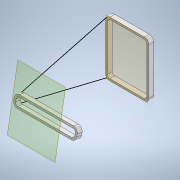
# Autodesk Inventor part: Rear Fan Shrowd
Saved by Autodesk Inventor 2020 (Build 240168000, 168)
## iProperties
Created: 2019-09-23
Part Number: Rear Fan Shrowd
Material: Generic
Document SubType Name: Modeling
Designer: pepd9
Density: 1 g/cm^3
Appearance: Default
Author: pepd9
Autodesk Inventor part; units mm, degrees
ref_plane "YZ Plane" through (0, 0, 0) normal (1, 0, 0) x (0, 1, 0)
ref_plane "XZ Plane" through (0, 0, 0) normal (0, 1, 0) x (-1, 0, 0)
ref_plane "XY Plane" through (0, 0, 0) normal (0, 0, 1) x (1, 0, 0)
ref_plane "Work Plane1" through (0, 0, 0) normal (0, 0, 1) x (1, 0, 0)
sketch "Sketch1" plane through (0, 0, 0) normal (0, 0, 1) x (1, 0, 0)
  line L0 (15.4, -2) -> (15.4, -18.2) projected
  arc A0 (15.4, -2) -> (13.4, 0) centre (13.4, -2) ccw projected
  line L1 (2, 0) -> (13.4, 0) projected
  arc A1 (2, 0) -> (0, -2) centre (2, -2) ccw projected
  line L2 (0, -18.2) -> (0, -2) projected
  arc A2 (0, -18.2) -> (2, -20.2) centre (2, -18.2) ccw projected
  line L3 (2, -20.2) -> (13.4, -20.2) projected
  arc A3 (13.4, -20.2) -> (15.4, -18.2) centre (13.4, -18.2) ccw projected
  arc A4 (1, -18.2) -> (2, -19.2) centre (2, -18.2) ccw projected
  line L4 (1, -2) -> (1, -18.2) projected
  arc A5 (2, -1) -> (1, -2) centre (2, -2) ccw projected
  line L5 (2, -1) -> (13.4, -1) projected
  arc A6 (14.4, -2) -> (13.4, -1) centre (13.4, -2) ccw projected
  line L6 (14.4, -2) -> (14.4, -18.2) projected
  arc A7 (13.4, -19.2) -> (14.4, -18.2) centre (13.4, -18.2) ccw projected
  line L7 (2, -19.2) -> (13.4, -19.2) projected
  line L8 (0.7, -20.5) -> (14.7, -20.5)
  line L9 (15.7, -19.5) -> (15.7, -0.7)
  line L10 (14.7, 0.3) -> (0.7, 0.3)
  line L11 (-0.3, -0.7) -> (-0.3, -19.5)
  arc A8 (0.7, 0.3) -> (-0.3, -0.7) centre (0.7, -0.7) ccw
  arc A9 (15.7, -0.7) -> (14.7, 0.3) centre (14.7, -0.7) ccw
  arc A10 (14.7, -20.5) -> (15.7, -19.5) centre (14.7, -19.5) ccw
  arc A11 (-0.3, -19.5) -> (0.7, -20.5) centre (0.7, -19.5) ccw
  line L12 (-1.1, -19.5) -> (-1.1, -0.7)
  arc A12 (0.7, 1.1) -> (-1.1, -0.7) centre (0.7, -0.7) ccw
  line L13 (0.7, 1.1) -> (14.7, 1.1)
  arc A13 (16.5, -0.7) -> (14.7, 1.1) centre (14.7, -0.7) ccw
  line L14 (16.5, -0.7) -> (16.5, -19.5)
  arc A14 (14.7, -21.3) -> (16.5, -19.5) centre (14.7, -19.5) ccw
  line L15 (14.7, -21.3) -> (0.7, -21.3)
  arc A15 (-1.1, -19.5) -> (0.7, -21.3) centre (0.7, -19.5) ccw
  dimension "d2" = 0.3
  dimension "d3" = 0.3
  dimension "d4" = 0.3
  dimension "d5" = 0.3
  dimension "d6" = 1
  dimension "d7" = 0.8
  constraints: 16 end point, 16 point on circle, 8 centre point, 8 tangent, 4 parallel, 3 equal radius, 2 perpendicular, 1 horizontal, 7 other
  measures "d2" distance between parallel lines of L1 L10
  measures "d3" distance between parallel lines of L8 L3
  measures "d4" distance between parallel lines of L11 L2
  measures "d5" distance between parallel lines of L9 L0
  measures "d6" radius of A8
  measures "d7" distance between parallel lines of L11 L12
extrude "Extrusion1" add sketch "Sketch1" against normal blind 2 contours L0 A3 L3 A2 L2 A1 L1 A0 | L4 A5 L5 A6 L6 A7 L7 A4 | A11 L11 A8 L10 A9 L9 A10 L8 | L12 A12 L13 A13 L14 A14 L15 A15
ref_plane "Work Plane3" through (18.9, -7.5485, 36.339) normal (0, -0.1736482, -0.9848078) x (-1, 0, 0)
sketch "Sketch2" plane through (18.9, -7.5485, 36.339) normal (0, -0.1736482, -0.9848078) x (-1, 0, 0)
  ellipse E0 centre (7.5, -3.3041) end of major axis (7.7, -3.3041) minor radius 0.0347 projected
  line L0 (-3.5, -1.3041) -> (18.5, -1.3041)
  line L1 (19.5, -2.3041) -> (19.5, -3.3041)
  line L2 (18.5, -4.3041) -> (-3.5, -4.3041)
  line L3 (-4.5, -3.3041) -> (-4.5, -2.3041)
  arc A0 (-3.5, -1.3041) -> (-4.5, -2.3041) centre (-3.5, -2.3041) ccw
  arc A1 (-4.5, -3.3041) -> (-3.5, -4.3041) centre (-3.5, -3.3041) ccw
  arc A2 (18.5, -4.3041) -> (19.5, -3.3041) centre (18.5, -3.3041) ccw
  arc A3 (19.5, -2.3041) -> (18.5, -1.3041) centre (18.5, -2.3041) ccw
  line L4 (18.5, -0.5041) -> (-3.5, -0.5041)
  arc A4 (-3.5, -0.5041) -> (-5.3, -2.3041) centre (-3.5, -2.3041) ccw
  line L5 (-5.3, -2.3041) -> (-5.3, -3.3041)
  arc A5 (-5.3, -3.3041) -> (-3.5, -5.1041) centre (-3.5, -3.3041) ccw
  line L6 (-3.5, -5.1041) -> (18.5, -5.1041)
  arc A6 (18.5, -5.1041) -> (20.3, -3.3041) centre (18.5, -3.3041) ccw
  line L7 (20.3, -3.3041) -> (20.3, -2.3041)
  arc A7 (20.3, -2.3041) -> (18.5, -0.5041) centre (18.5, -2.3041) ccw
  point P0 (18.9, 13.744)
  dimension "d11" = 12
  dimension "d12" = 12
  dimension "d13" = 2
  dimension "d14" = 1
  dimension "d15" = 1
  dimension "d16" = 0.8
  constraints: 16 end point, 16 point on circle, 8 centre point, 8 tangent, 4 parallel, 3 equal radius, 2 perpendicular, 1 horizontal, 7 other
  measures "d11" distance from line of L3 E0.centre
  measures "d12" distance from line of L1 E0.centre
  measures "d13" distance from line of E0.centre L0
  measures "d14" distance from line of L2 E0.centre
  measures "d15" radius of A0
  measures "d16" distance between parallel lines of L0 L4
extrude "Extrusion2" add sketch "Sketch2" along normal blind 2 contours L0 A3 L1 A2 L2 A1 L3 A0 | A7 L7 A6 L6 A5 L5 A4 L4
sketch3d "3D Sketch1"
sketch "Sketch3" plane through (0, 0, 0) normal (0, 0, 1) x (1, 0, 0)
  line L0 (14.7, 1.1) -> (0.7, 1.1) projected
  arc A0 (0.7, 1.1) -> (-1.1, -0.7) centre (0.7, -0.7) ccw projected
  line L1 (-1.1, -0.7) -> (-1.1, -19.5) projected
  arc A1 (-1.1, -19.5) -> (0.7, -21.3) centre (0.7, -19.5) ccw projected
  line L2 (0.7, -21.3) -> (14.7, -21.3) projected
  arc A2 (14.7, -21.3) -> (16.5, -19.5) centre (14.7, -19.5) ccw projected
  line L3 (16.5, -19.5) -> (16.5, -0.7) projected
  arc A3 (16.5, -0.7) -> (14.7, 1.1) centre (14.7, -0.7) ccw projected
  point P0 (0, 0)
sketch "Sketch4" plane through (18.9, -7.8958, 34.3694) normal (0, -0.1736482, -0.9848078) x (-1, 0, 0)
  line L0 (20.3, -3.3041) -> (20.3, -2.3041) projected
  arc A0 (20.3, -2.3041) -> (18.5, -0.5041) centre (18.5, -2.3041) ccw projected
  line L1 (18.5, -0.5041) -> (-3.5, -0.5041) projected
  arc A1 (-3.5, -0.5041) -> (-5.3, -2.3041) centre (-3.5, -2.3041) ccw projected
  line L2 (-5.3, -2.3041) -> (-5.3, -3.3041) projected
  arc A2 (-5.3, -3.3041) -> (-3.5, -5.1041) centre (-3.5, -3.3041) ccw projected
  line L3 (-3.5, -5.1041) -> (18.5, -5.1041) projected
  arc A3 (18.5, -5.1041) -> (20.3, -3.3041) centre (18.5, -3.3041) ccw projected
  point P0 (18.9, 13.744)
body "Solid1"
